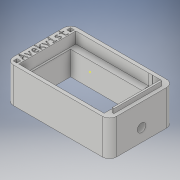
# Autodesk Inventor part: AttendMiddle
Saved by Autodesk Inventor 2019 (Build 230136000, 136)
## iProperties
Created: 2018-11-13
Part Number: AttendMiddle
Material: Generic
Document SubType Name: Modeling
Designer: hampu
Density: 1 g/cm^3
Appearance: Default
Author: hampu
Autodesk Inventor part; units mm, degrees
ref_plane "YZ Plane" through (0, 0, 0) normal (1, 0, 0) x (0, 1, 0)
ref_plane "XZ Plane" through (0, 0, 0) normal (0, 1, 0) x (-1, 0, 0)
ref_plane "XY Plane" through (0, 0, 0) normal (0, 0, 1) x (1, 0, 0)
sketch "Sketch1" plane through (0, 0, 0) normal (0, 1, 0) x (-1, 0, 0)
  line L0 (36.595, -22.775) -> (-36.595, -22.775)
  line L1 (-36.595, -22.775) -> (-36.595, 22.775)
  line L2 (-36.595, 22.775) -> (36.595, 22.775)
  line L3 (36.595, 22.775) -> (36.595, -22.775)
  line L4 (36.595, -22.775) -> (-36.595, 22.775) construction
  line L5 (-36.595, -22.775) -> (36.595, 22.775) construction
  line L6 (34.195, -17.675) -> (31.495, -17.675)
  line L7 (31.495, -17.675) -> (31.495, -20.375)
  line L8 (31.495, -20.375) -> (34.195, -20.375)
  line L9 (34.195, -20.375) -> (34.195, -17.675)
  line L10 (-24.195, -17.675) -> (-21.495, -17.675)
  line L11 (-21.495, -17.675) -> (-21.495, -20.375)
  line L12 (-21.495, -20.375) -> (-24.195, -20.375)
  line L13 (-24.195, -20.375) -> (-24.195, -17.675)
  line L14 (-21.495, 20.375) -> (-24.195, 20.375)
  line L15 (-24.195, 20.375) -> (-24.195, 17.675)
  line L16 (-24.195, 17.675) -> (-21.495, 17.675)
  line L17 (-21.495, 17.675) -> (-21.495, 20.375)
  line L18 (31.495, 20.375) -> (34.195, 20.375)
  line L19 (34.195, 20.375) -> (34.195, 17.675)
  line L20 (34.195, 17.675) -> (31.495, 17.675)
  line L21 (31.495, 17.675) -> (31.495, 20.375)
  line L22 (28.995, -15.175) -> (-18.995, -15.175)
  line L23 (-18.995, -15.175) -> (-18.995, 15.175)
  line L24 (-18.995, 15.175) -> (28.995, 15.175)
  line L25 (28.995, 15.175) -> (28.995, -15.175)
  line L26 (-18.995, 15.175) -> (-31.595, 15.175)
  line L27 (-31.595, 15.175) -> (-31.595, -15.175)
  line L28 (-31.595, -15.175) -> (-18.995, -15.175)
  line L29 (-18.995, -15.175) -> (-18.995, 15.175)
  line L30 (34.195, 20.375) -> (-24.195, 20.375)
  line L31 (-24.195, 20.375) -> (-24.195, 17.675)
  line L32 (-24.195, 17.675) -> (34.195, 17.675)
  line L33 (34.195, 17.675) -> (34.195, 20.375)
  line L34 (34.195, -17.675) -> (-24.195, -17.675)
  line L35 (-24.195, -17.675) -> (-24.195, -20.375)
  line L36 (-24.195, -20.375) -> (34.195, -20.375)
  line L37 (34.195, -20.375) -> (34.195, -17.675)
  point P0 (0, 0)
  dimension "d0" = 73.19
  dimension "d1" = 45.55
  dimension "d12" = 47.99
  dimension "d13" = 30.35
  dimension "d14" = 12.6
  constraints: 76 end point, 18 parallel, 9 perpendicular, 5 horizontal, 2 midpoint, 1 point on line
  measures "d0" distance of L1.end L2.end
  measures "d1" distance of L0.end L1.end
  measures "d12" distance of L23.end L24.end
  measures "d13" distance of L22.end L23.end
  measures "d14" distance of L28.end L27.end
extrude "Extrusion1" add sketch "Sketch1" along normal blind 25 contours L0 L1 L2 L3 | L7 L36 L11 L34 | L30 L21 L32 L17
sketch "Sketch4" plane through (0, 25, 0) normal (0, 1, 0) x (1, 0, 0)
  line L0 (-30, 20) -> (30, -20) construction
  line L1 (30, 20) -> (-30, -20) construction
  line L2 (30.3, 20.3) -> (-30.3, 20.3)
  line L3 (-30.3, 20.3) -> (-30.3, -20.3)
  line L4 (-30.3, -20.3) -> (30.3, -20.3)
  line L5 (30.3, -20.3) -> (30.3, 20.3)
  point P0 (0, 0)
  dimension "d21" = 60
  dimension "d22" = 40
  constraints: 12 end point, 2 midpoint, 2 parallel, 1 perpendicular
  measures "d21" distance of L0.end L1.end
  measures "d22" distance of L1.start L0.end
extrude "Extrusion2" cut sketch "Sketch4" against normal blind 8
sketch "Sketch6" plane through (0, 25, 0) normal (0, 1, 0) x (1, 0, 0)
  line L0 (-31.495, -17.675) -> (-34.195, -17.675) projected
  line L1 (-31.495, 20.375) -> (-31.495, 17.675) projected
  line L2 (-34.195, -17.675) -> (-31.495, -17.675)
  line L3 (-31.495, -17.675) -> (-31.495, 17.675)
  line L4 (-31.495, 17.675) -> (-34.195, 17.675)
  line L5 (-34.195, 17.675) -> (-34.195, -17.675)
  line L6 (-35.995, -14.0801) -> (-30.995, -12.6012)
  line L7 (-30.995, -12.6012) -> (-30.995, -13.2614)
  line L8 (-30.995, -13.2614) -> (-32.6103, -13.7368)
  line L9 (-32.6103, -13.7368) -> (-32.6103, -15.1408)
  line L10 (-32.6103, -15.1408) -> (-30.995, -15.6118)
  line L11 (-30.995, -15.6118) -> (-30.995, -16.2676)
  line L12 (-30.995, -16.2676) -> (-35.995, -14.7931)
  line L13 (-35.995, -14.7931) -> (-35.995, -14.0801)
  line L14 (-33.1121, -15.0088) -> (-33.1121, -13.8644)
  line L15 (-33.1121, -13.8644) -> (-35.282, -14.4278)
  line L16 (-35.282, -14.4278) -> (-33.1121, -15.0088)
  spline S0 degree 2 poles (-31.6288, -10.2993) (-32.4255, -10.0088) (-34.6746, -9.221) knots 0 0 0 1 1 1
  line L17 (-34.6746, -9.221) -> (-34.6746, -8.5431)
  line L18 (-34.6746, -8.5431) -> (-30.995, -9.978)
  line L19 (-30.995, -9.978) -> (-30.995, -10.6602)
  line L20 (-30.995, -10.6602) -> (-34.6746, -12.0819)
  line L21 (-34.6746, -12.0819) -> (-34.6746, -11.3776)
  line L22 (-34.6746, -11.3776) -> (-31.6288, -10.2993)
  spline S1 degree 2 poles (-31.1667, -6.875) (-31.4263, -7.2623) (-32.2934, -7.6364) (-33.385, -7.6364) (-34.2564, -7.2887) (-34.789, -6.6021) (-34.789, -6.1884) knots 0 0 0 1 2 3 4 5 5 5
  spline S2 degree 2 poles (-34.789, -6.1884) (-34.789, -5.4093) (-33.7239, -4.6875) (-32.9448, -4.6875) knots 0 0 0 1 2 2 2
  line L23 (-32.9448, -4.6875) -> (-32.738, -4.6875)
  line L24 (-32.738, -4.6875) -> (-32.738, -7.0158)
  spline S3 degree 2 poles (-32.738, -7.0158) (-32.1746, -6.9982) (-31.3823, -6.4701) (-31.3823, -5.9419) knots 0 0 0 1 2 2 2
  spline S4 degree 2 poles (-31.3823, -5.9419) (-31.4131, -5.5898) (-31.7652, -4.9604) knots 0 0 0 1 1 1
  line L25 (-31.7652, -4.9604) -> (-31.3471, -4.7579)
  spline S5 degree 2 poles (-31.3471, -4.7579) (-30.9114, -5.1937) (-30.9114, -5.9507) knots 0 0 0 1 1 1
  spline S6 degree 2 poles (-30.9114, -5.9507) (-30.9114, -6.4921) (-31.1667, -6.875) knots 0 0 0 1 1 1
  spline S7 degree 2 poles (-33.1869, -5.2685) (-34.3181, -5.3345) (-34.3181, -6.0607) knots 0 0 0 1 1 1
  spline S8 degree 2 poles (-34.3181, -6.0607) (-34.3181, -6.8794) (-33.1869, -6.9982) knots 0 0 0 1 1 1
  line L26 (-33.1869, -6.9982) -> (-33.1869, -5.2685)
  line L27 (-33.1825, -2.8081) -> (-34.6746, -1.1796)
  line L28 (-34.6746, -1.1796) -> (-34.6746, -0.4049)
  line L29 (-34.6746, -0.4049) -> (-33.1473, -2.0467)
  line L30 (-33.1473, -2.0467) -> (-30.995, -0.1805)
  line L31 (-30.995, -0.1805) -> (-30.995, -0.9463)
  line L32 (-30.995, -0.9463) -> (-32.8656, -2.4824)
  line L33 (-32.8656, -2.4824) -> (-32.5795, -2.8081)
  line L34 (-32.5795, -2.8081) -> (-30.995, -2.8081)
  line L35 (-30.995, -2.8081) -> (-30.995, -3.4199)
  line L36 (-30.995, -3.4199) -> (-36.1799, -3.4199)
  line L37 (-36.1799, -3.4199) -> (-36.2459, -2.8081)
  line L38 (-36.2459, -2.8081) -> (-33.1825, -2.8081)
  spline S9 degree 2 poles (-31.6288, 2.0731) (-32.4255, 2.3636) (-34.6746, 3.1514) knots 0 0 0 1 1 1
  line L39 (-34.6746, 3.1514) -> (-34.6746, 3.8292)
  line L40 (-34.6746, 3.8292) -> (-30.995, 2.3944)
  line L41 (-30.995, 2.3944) -> (-30.995, 1.7121)
  line L42 (-30.995, 1.7121) -> (-34.6746, 0.2905)
  line L43 (-34.6746, 0.2905) -> (-34.6746, 0.9947)
  line L44 (-34.6746, 0.9947) -> (-31.6288, 2.0731)
  line L45 (-34.2036, 4.978) -> (-34.6746, 4.978)
  line L46 (-34.6746, 4.978) -> (-34.6746, 6.6417)
  line L47 (-34.6746, 6.6417) -> (-31.466, 6.6417)
  line L48 (-31.466, 6.6417) -> (-31.466, 7.6937)
  line L49 (-31.466, 7.6937) -> (-30.995, 7.6937)
  line L50 (-30.995, 7.6937) -> (-30.995, 4.8636)
  line L51 (-30.995, 4.8636) -> (-31.466, 4.8636)
  line L52 (-31.466, 4.8636) -> (-31.466, 6.0299)
  line L53 (-31.466, 6.0299) -> (-34.2036, 6.0299)
  line L54 (-34.2036, 6.0299) -> (-34.2036, 4.978)
  line L55 (-35.6429, 5.9287) -> (-35.9774, 5.9287)
  spline S10 degree 2 poles (-35.9774, 5.9287) (-36.0962, 5.9287) (-36.2811, 6.2016) (-36.2811, 6.4701) (-36.0962, 6.743) (-35.9774, 6.743) knots 0 0 0 1 2 3 4 4 4
  line L56 (-35.9774, 6.743) -> (-35.6429, 6.743)
  spline S11 degree 2 poles (-35.6429, 6.743) (-35.524, 6.743) (-35.3392, 6.4701) (-35.3392, 6.2016) (-35.524, 5.9287) (-35.6429, 5.9287) knots 0 0 0 1 2 3 4 4 4
  spline S12 degree 2 poles (-33.0857, 10.757) (-32.9668, 11.2324) (-32.4563, 11.6725) (-31.4968, 11.6725) (-30.9114, 10.9375) (-30.9114, 10.3873) knots 0 0 0 1 2 3 4 4 4
  spline S13 degree 2 poles (-30.9114, 10.3873) (-30.9114, 9.9912) (-31.1094, 9.243) (-31.2415, 9.0669) knots 0 0 0 1 2 2 2
  line L57 (-31.2415, 9.0669) -> (-31.6816, 9.2165)
  spline S14 degree 2 poles (-31.6816, 9.2165) (-31.5936, 9.3574) (-31.4175, 9.9692) (-31.4175, 10.6822) (-31.7168, 11.1092) (-32.2142, 11.1092) (-32.4959, 10.8979) (-32.5707, 10.5986) knots 0 0 0 1 2 3 4 5 6 6 6
  line L58 (-32.5707, 10.5986) -> (-32.7248, 9.9736)
  spline S15 degree 2 poles (-32.7248, 9.9736) (-32.8568, 9.4322) (-33.3718, 9.0757) (-34.1332, 9.0757) (-34.7802, 9.6963) (-34.7846, 10.2905) knots 0 0 0 1 2 3 4 4 4
  line L59 (-34.7846, 10.2905) -> (-34.7846, 10.3345)
  spline S16 degree 2 poles (-34.7846, 10.3345) (-34.7846, 11.0035) (-34.5337, 11.4701) knots 0 0 0 1 1 1
  line L60 (-34.5337, 11.4701) -> (-34.1068, 11.338)
  spline S17 degree 2 poles (-34.1068, 11.338) (-34.3137, 10.8495) (-34.3137, 10.3433) knots 0 0 0 1 1 1
  spline S18 degree 2 poles (-34.3137, 10.3433) (-34.3093, 10.0352) (-34.0056, 9.6347) (-33.5434, 9.6347) (-33.3101, 9.8371) (-33.2441, 10.1188) knots 0 0 0 1 2 3 4 4 4
  line L61 (-33.2441, 10.1188) -> (-33.0857, 10.757)
  line L62 (-34.2036, 14.3266) -> (-32.4783, 14.3266)
  spline S19 degree 2 poles (-32.4783, 14.3266) (-32.157, 14.3266) (-31.7785, 14.397) (-31.5452, 14.6083) (-31.466, 14.9472) (-31.466, 15.2333) knots 0 0 0 1 2 3 4 4 4
  line L63 (-31.466, 15.2333) -> (-31.466, 15.9067)
  line L64 (-31.466, 15.9067) -> (-30.995, 15.8759)
  line L65 (-30.995, 15.8759) -> (-30.995, 15.2597)
  spline S20 degree 2 poles (-30.995, 15.2597) (-30.995, 14.309) (-31.3427, 13.9921) knots 0 0 0 1 1 1
  spline S21 degree 2 poles (-31.3427, 13.9921) (-31.5716, 13.7896) (-32.0777, 13.7412) knots 0 0 0 1 1 1
  spline S22 degree 2 poles (-32.0777, 13.7412) (-32.3022, 13.7192) (-32.6323, 13.7192) knots 0 0 0 1 1 1
  line L66 (-32.6323, 13.7192) -> (-34.2036, 13.7192)
  line L67 (-34.2036, 13.7192) -> (-34.2036, 12.6761)
  line L68 (-34.2036, 12.6761) -> (-34.6746, 12.7465)
  line L69 (-34.6746, 12.7465) -> (-34.6746, 13.7192)
  line L70 (-34.6746, 13.7192) -> (-35.9422, 13.7192)
  line L71 (-35.9422, 13.7192) -> (-36.1226, 14.3266)
  line L72 (-36.1226, 14.3266) -> (-34.6746, 14.3266)
  line L73 (-34.6746, 14.3266) -> (-34.6746, 15.8803)
  line L74 (-34.6746, 15.8803) -> (-34.2036, 15.8803)
  line L75 (-34.2036, 15.8803) -> (-34.2036, 14.3266)
  point P0 (0, 0)
  constraints: 8 end point, 2 parallel, 1 horizontal, 1 perpendicular, 1 vertical
extrude "Extrusion4" cut sketch "Sketch6" against normal blind 2 contours L12 L5 L16 L14 L15 L6 L3 L8 L9 L10 | L3 L10 L11 L12 | L12 L13 L6 L5 L15 L16 | L3 L6 L7 L8 | L20 L5 L22 S0 L18 L3 | L3 L18 L19 L20 | L20 L21 L22 L5 | S1 L5 S8 L26 S7 S2 L23 L24 S3 L3 | L3 S3 S4 L25 S5 S6 S1 | L5 S0 L17 L18 | S1 S2 L5 S7 S8 | S4 L25 L3 | L36 L5 L38 L27 L29 L30 L3 L32 L33 L34 | L3 L34 L35 L36 | L36 L37 L38 L5 | L3 L30 L31 L32 | L27 L28 L29 L5 | L42 L5 L44 S9 L40 L3 | L3 L40 L41 L42 | L42 L43 L44 L5 | L53 L5 L47 L3 | L3 L47 L48 L49 L50 L51 L52 L53 | L5 S9 L39 L40 | L53 L54 L45 L46 L47 L5 | L57 S14 L3 | L3 S14 S12 S13 L57 | S15 L59 S16 L60 L5 S17 S18 | L5 S18 L61 S12 L3 S14 L58 S15 | L5 L60 S17 | S21 S22 L66 L5 L62 S19 L3 | L3 S19 L63 L64 L65 S20 S21 | L66 L67 L68 L69 L70 L71 L72 L73 L74 L75 L62 L5 | L55 S10 L56 S11
fillet "Fillet1" radius 5 4 edges at (36.595, 12.5, -22.775) (36.595, 12.5, 22.775) (-36.595, 12.5, -22.775) (-36.595, 12.5, 22.775)
sketch "Sketch7" plane through (36.595, 0, 17.775) normal (1, 0, 0) x (0, 0, -1)
  line L0 (12.775, 14.1349) -> (22.775, 14.1349)
  line L1 (22.775, 14.1349) -> (22.775, 4.1349)
  line L2 (22.775, 4.1349) -> (12.775, 4.1349)
  line L3 (12.775, 4.1349) -> (12.775, 14.1349)
  line L4 (12.775, 14.1349) -> (22.775, 4.1349) construction
  line L5 (22.775, 14.1349) -> (12.775, 4.1349) construction
  circle A0 centre (17.775, 9.1349) radius 3
  point P0 (17.775, 0)
  dimension "d37" = 10
  dimension "d38" = 10
  dimension "d39" = 6
  constraints: 12 end point, 2 midpoint, 2 parallel, 1 centre point, 1 coincident, 1 horizontal, 1 perpendicular
  measures "d37" distance of L1.end L2.end
  measures "d38" distance of L0.end L1.end
  measures "d39" diameter of A0
extrude "Extrusion5" cut sketch "Sketch7" against normal blind 5 contours A0
sketch "Sketch8" plane through (0, 0, 0) normal (0, -1, 0) x (1, 0, 0)
  line L0 (-31.495, 20.375) -> (21.495, 20.375)
  line L1 (21.495, 20.375) -> (21.495, 17.675)
  line L2 (21.495, 17.675) -> (-31.495, 17.675)
  line L3 (-31.495, 17.675) -> (-31.495, 20.375)
  line L4 (21.495, -20.3) -> (21.495, -17.675) projected
  line L5 (21.495, -17.675) -> (-31.495, -17.675)
  line L6 (-31.495, -17.675) -> (-31.495, -20.3)
  line L7 (-31.495, -20.3) -> (21.495, -20.3)
  line L8 (21.495, -20.3) -> (21.495, -17.675)
  point P0 (0, 0)
  constraints: 16 end point, 4 parallel, 2 horizontal, 2 perpendicular, 1 point on line
extrude "Extrusion6" cut sketch "Sketch8" against normal blind 15
sketch "Sketch9" plane through (0, 25, 0) normal (0, 1, 0) x (1, 0, 0)
  line L0 (32.695, -17) -> (33.995, -17)
  line L1 (33.995, -17) -> (33.995, 17)
  line L2 (33.995, 17) -> (32.695, 17)
  line L3 (32.695, 17) -> (32.695, -17)
  line L4 (32.695, -17) -> (33.995, 17) construction
  line L5 (33.995, -17) -> (32.695, 17) construction
  point P0 (0, 0)
  point P1 (33.345, 0)
  dimension "d50" = 34
  constraints: 12 end point, 2 midpoint, 2 parallel, 1 horizontal, 1 perpendicular
  measures "d50" distance of L1.end L0.end
extrude "Extrusion7" add sketch "Sketch9" along normal blind 3
sketch "Sketch11" plane through (0, 25, 0) normal (0, 1, 0) x (1, 0, 0)
  point P0 (0, 0)
sketch "Sketch12" plane through (0, 0, 0) normal (0, -1, 0) x (1, 0, 0)
  point P0 (0, 0)
sketch "Sketch13" plane through (0, 25, 0) normal (0, 1, 0) x (1, 0, 0)
  point P0 (0, 0)
body "Solid1"
